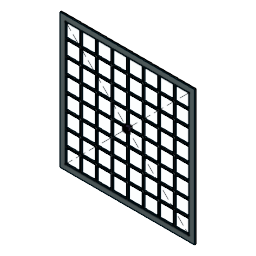
Atlas_Surface_Core_SC001 (Autodesk Fusion 360 design; units mm, degrees)
part number: 2026-07-13-13-13-09-945
Autodesk Fusion 360 part; units mm, degrees
sketch "Sketch1" plane through (0, 0, 0) normal (0, 0, 1) x (1, 0, 0)
  line L0 (120.65, 120.65) -> (-120.65, 120.65)
  line L1 (-120.65, 120.65) -> (-120.65, -120.65)
  line L2 (-120.65, -120.65) -> (120.65, -120.65)
  line L3 (120.65, -120.65) -> (120.65, 120.65)
  line L4 (120.65, 120.65) -> (-120.65, -120.65) construction
  line L5 (-120.65, 120.65) -> (120.65, -120.65) construction
  dimension "d10" = 241.3
  dimension "d11" = 241.3
  constraint horizontal L0
  constraint perpendicular L0 L1
  constraint parallel L0 L2
  constraint parallel L1 L3
  constraint coincident L4 origin
  constraint coincident L5 origin
  measures "d10" distance of L1.end L2.end
  measures "d11" distance of L0.end L1.end
extrude "Extrude1" add sketch "Sketch1" along normal blind 2.54
sketch "Sketch2" plane through (0, 0, 2.54) normal (0, 0, 1) x (1, 0, 0)
  line L0 (120.65, -120.65) -> (120.65, 120.65)
  line L1 (120.65, 120.65) -> (-120.65, 120.65)
  line L2 (-120.65, 120.65) -> (-120.65, -120.65)
  line L3 (-120.65, -120.65) -> (120.65, -120.65)
  line L4 (110.49, 110.49) -> (-110.49, 110.49)
  line L5 (-110.49, 110.49) -> (-110.49, -110.49)
  line L6 (-110.49, -110.49) -> (110.49, -110.49)
  line L7 (110.49, -110.49) -> (110.49, 110.49)
  line L8 (110.49, 110.49) -> (-110.49, -110.49) construction
  line L9 (-110.49, 110.49) -> (110.49, -110.49) construction
  dimension "d14" = 220.98
  dimension "d15" = 220.98
  constraint horizontal L4
  constraint perpendicular L4 L5
  constraint parallel L4 L6
  constraint parallel L5 L7
  constraint coincident L8 origin
  constraint coincident L9 origin
  measures "d14" distance of L5.end L6.end
  measures "d15" distance of L4.end L5.end
sketch "Sketch3" plane through (0, 0, 2.54) normal (0, 0, 1) x (1, 0, 0)
  line L0 (110.49, 110.49) -> (-110.49, 110.49)
  line L1 (110.49, -110.49) -> (110.49, 110.49)
  line L2 (-110.49, -110.49) -> (110.49, -110.49)
  line L3 (-110.49, 110.49) -> (-110.49, -110.49)
  line L4 (-110.49, 110.49) -> (-85.09, 110.49)
  line L5 (-85.09, 110.49) -> (-85.09, 85.09)
  line L6 (-85.09, 85.09) -> (-110.49, 85.09)
  line L7 (-110.49, 85.09) -> (-110.49, 110.49)
  dimension "d16" = 25.4
  dimension "d17" = 25.4
  constraint horizontal L4
  constraint vertical L5
  constraint horizontal L6
  constraint vertical L7
  constraint coincident L0.end L3.start
  measures "d16" distance of L0.end L4.end
  measures "d17" distance of L0.end L6.end
sketch "Sketch4" plane through (0, 0, 2.54) normal (0, 0, 1) x (1, 0, 0)
  line L0 (110.49, 110.49) -> (-110.49, 110.49)
  line L1 (110.49, -110.49) -> (110.49, 110.49)
  line L2 (-110.49, -110.49) -> (110.49, -110.49)
  line L3 (-110.49, 110.49) -> (-110.49, -110.49)
  line L4 (-110.49, 110.49) -> (-85.09, 110.49)
  line L5 (-85.09, 110.49) -> (-85.09, 85.09)
  line L6 (-85.09, 85.09) -> (-110.49, 85.09)
  line L7 (-110.49, 85.09) -> (-110.49, 110.49)
  dimension "d20" = 25.4
  dimension "d21" = 25.4
  constraint horizontal L4
  constraint vertical L5
  constraint horizontal L6
  constraint vertical L7
  constraint coincident L0.end L3.start
  measures "d20" distance of L0.end L4.end
  measures "d21" distance of L0.end L6.end
extrude "Grid First Cut" cut sketch "Sketch4" against normal blind 5.08 contours L0 L3 L4 L5 L6 L7
pattern_linear "R-Pattern1" count 8 spacing 27.94 along (1, 0, 0) count 8 spacing 27.94 along (0, -1, 0) of "Grid First Cut"
extrude "Extrude2" [rolled back] along distance -5.08 taper angle 0
equation "surfaceWidth = 9.5 in"
equation "surfaceDepth = 9.5 in"
equation "surfaceThickness = 0.1 in"
equation "borderWidth = 0.4 in"
equation "gridOpeningX = 1 in"
equation "gridOpeningY = 1 in"
equation "gridWebWidth = 0.1 in"
equation "payloadWidth = surfaceWidth - ( 2 * borderWidth )"
equation "payloadDepth = surfaceDepth - ( 2 * borderWidth )"
equation "d10 = surfaceWidth"
equation "d11 = surfaceDepth"
equation "d12 = surfaceThickness"
equation "d14 = payloadWidth"
equation "d15 = payloadDepth"
equation "d16 = gridOpeningX"
equation "d17 = gridOpeningY"
equation "d20 = gridOpeningY"
equation "d21 = gridOpeningX"
equation "gridCountX = 8"
equation "gridCountY = 8"
equation "gridPitchX = gridOpeningX + gridWebWidth"
equation "d27 = gridCountY"
equation "d28 = gridCountY"
equation "d29 = gridPitchX"
equation "d30 = gridPitchX"
